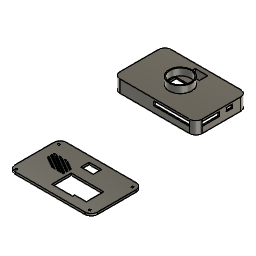
Camra_V1 v1 (Autodesk Fusion 360 design; units mm, degrees)
Autodesk Fusion 360 part; units mm, degrees
sketch "Boceto1" plane through (0, 0, 0) normal (0, 0, 1) x (1, 0, 0)
  line L0 (7, 0) -> (108, 0)
  line L1 (0, -7) -> (0, -63)
  line L2 (7, -70) -> (108, -70)
  line L3 (115, -63) -> (115, -7)
  arc A0 (7, 0) -> (0, -7) centre (7, -7) ccw
  arc A1 (0, -63) -> (7, -70) centre (7, -63) ccw
  arc A2 (108, -70) -> (115, -63) centre (108, -63) ccw
  arc A3 (115, -7) -> (108, 0) centre (108, -7) ccw
  line L4 (67.5, -3.5) -> (47.5, -3.5)
  line L5 (47.5, -3.5) -> (47.5, -17.5)
  line L6 (47.5, -17.5) -> (67.5, -17.5)
  line L7 (67.5, -17.5) -> (67.5, -3.5)
  circle A4 centre (4.1716, -4.1716) radius 2
  circle A5 centre (4.1716, -65.8284) radius 2
  circle A6 centre (108.8284, -63.8284) radius 2
  circle A7 centre (110.8284, -4.1716) radius 2
  line L8 (48.5, -4.5) -> (48.5, -16.5)
  line L9 (48.5, -16.5) -> (66.5, -16.5)
  line L10 (66.5, -16.5) -> (66.5, -4.5)
  line L11 (66.5, -4.5) -> (48.5, -4.5)
  arc A8 (117, -7) -> (108, 2) centre (108, -7) ccw
  line L12 (7, 2) -> (108, 2)
  arc A9 (7, 2) -> (-2, -7) centre (7, -7) ccw
  line L13 (-2, -7) -> (-2, -63)
  arc A10 (-2, -63) -> (7, -72) centre (7, -63) ccw
  line L14 (7, -72) -> (108, -72)
  arc A11 (108, -72) -> (117, -63) centre (108, -63) ccw
  line L15 (117, -63) -> (117, -7)
  arc A12 (0, -164.4825) -> (7, -171.4825) centre (7, -164.4825) ccw
  line L16 (66.5, -107.9825) -> (48.5, -107.9825)
  arc A13 (117, -108.4825) -> (108, -99.4825) centre (108, -108.4825) ccw
  circle A14 centre (108.8284, -167.311) radius 1.5
  circle A15 centre (110.8284, -107.6541) radius 1.5
  arc A16 (-2, -164.4825) -> (7, -173.4825) centre (7, -164.4825) ccw
  line L17 (48.5, -119.9825) -> (66.5, -119.9825)
  line L18 (67.5, -120.9825) -> (67.5, -106.9825)
  line L19 (67.5, -106.9825) -> (47.5, -106.9825)
  line L20 (47.5, -120.9825) -> (67.5, -120.9825)
  line L21 (47.5, -106.9825) -> (47.5, -120.9825)
  line L22 (7, -173.4825) -> (108, -173.4825)
  line L23 (7, -101.4825) -> (108, -101.4825)
  line L24 (7, -171.4825) -> (108, -171.4825)
  line L25 (-2, -108.4825) -> (-2, -164.4825)
  line L26 (0, -108.4825) -> (0, -164.4825)
  arc A17 (115, -108.4825) -> (108, -101.4825) centre (108, -108.4825) ccw
  circle A18 centre (4.1716, -169.311) radius 1.5
  arc A19 (108, -171.4825) -> (115, -164.4825) centre (108, -164.4825) ccw
  line L27 (115, -164.4825) -> (115, -108.4825)
  arc A20 (7, -99.4825) -> (-2, -108.4825) centre (7, -108.4825) ccw
  line L28 (48.5, -107.9825) -> (48.5, -119.9825)
  arc A21 (7, -101.4825) -> (0, -108.4825) centre (7, -108.4825) ccw
  arc A22 (108, -173.4825) -> (117, -164.4825) centre (108, -164.4825) ccw
  circle A23 centre (4.1716, -107.6541) radius 1.5
  line L29 (66.5, -119.9825) -> (66.5, -107.9825)
  line L30 (117, -164.4825) -> (117, -108.4825)
  line L31 (7, -99.4825) -> (108, -99.4825)
  circle A24 centre (57.5, -35) radius 16.5
  circle A25 centre (57.5, -35) radius 15
  line L32 (57.5, -29) -> (57.0394, -29)
  line L33 (57.5, -29) -> (58, -29)
  line L34 (58, -29) -> (68.4659, -29)
  line L35 (57.5, -29) -> (46.5341, -29)
  line L36 (57.5, -41) -> (68.4659, -41)
  line L37 (57.5, -41) -> (46.5341, -41)
  arc A26 (46.5341, -41) -> (68.4659, -41) centre (57.5, -35) ccw
  arc A27 (68.4659, -29) -> (46.5341, -29) centre (57.5, -35) ccw
  line L38 (68.4659, -29) -> (68.4659, -41)
  line L39 (46.5341, -29) -> (46.5341, -41)
  circle A28 centre (57.5, -35) radius 12.5081
  line L40 (12, -125) -> (40, -141)
  line L41 (12, -123) -> (43, -141)
  line L42 (15, -122) -> (44, -138.8387)
  line L43 (18.983, -122) -> (44, -136.526)
  line L44 (22.966, -122) -> (44, -134.2133)
  line L45 (12, -127.3035) -> (35.9689, -141)
  line L46 (12, -129.607) -> (31.9377, -141)
  line L47 (12, -131.9105) -> (27.9066, -141)
  line L48 (26.949, -122) -> (44, -131.9006)
  line L49 (12, -131.9105) -> (12, -129.607)
  line L50 (31.9377, -141) -> (27.9066, -141)
  line L51 (12, -127.3035) -> (12, -125)
  line L52 (12, -123) -> (12, -122)
  line L53 (44, -141) -> (43, -141)
  line L54 (40, -141) -> (35.9689, -141)
  line L55 (12, -122) -> (15, -122)
  line L56 (44, -138.8387) -> (44, -141)
  line L57 (44, -134.2133) -> (44, -136.526)
  line L58 (18.983, -122) -> (22.966, -122)
  line L59 (34.3764, -124) -> (42, -128.4266)
  line L60 (34.3764, -124) -> (30.932, -122)
  line L61 (42, -128.4266) -> (44, -129.5879)
  line L62 (30.932, -122) -> (26.949, -122)
  line L63 (44, -129.5879) -> (44, -131.9006)
  point P0 (115, 0)
  point P1 (0, -70)
  point P2 (0, -101.4825)
  point P3 (0, -101.4825)
  point P4 (0, -101.4825)
  point P5 (115, -101.4825)
  point P6 (0, -171.4825)
  dimension "d1" = 115
  dimension "d2" = 70
  dimension "d8" = 7
  dimension "d9" = 7
  dimension "d10" = 7
  dimension "d11" = 7
  dimension "d20" = 14
  dimension "d25" = 4
  dimension "d27" = 4
  dimension "d29" = 4
  dimension "d31" = 4
  dimension "d32" = -1
  dimension "d33" = -2
  dimension "d34" = -1
  dimension "d35" = -2
  dimension "d36" = 115
  dimension "d37" = 70
  dimension "d38" = 7
  dimension "d39" = 7
  dimension "d40" = 7
  dimension "d41" = 7
  dimension "d46" = 14
  dimension "d47" = 3
  dimension "d48" = 3
  dimension "d49" = 3
  dimension "d50" = 3
  dimension "d63" = 33
  dimension "d65" = 25
  constraint horizontal L0
  constraint perpendicular L0 L1
  constraint perpendicular L1 L2
  constraint perpendicular L0 L3
  constraint coincident origin L1
  constraint coincident origin L0
  constraint tangent L1 A0
  constraint tangent L0 A0
  constraint coincident P1 L2
  constraint coincident P1 L1
  constraint tangent L2 A1
  constraint tangent L1 A1
  constraint tangent L3 A2
  constraint tangent L2 A2
  constraint coincident P0 L3
  constraint coincident P0 L0
  constraint tangent L3 A3
  constraint tangent L0 A3
  constraint horizontal L4
  constraint vertical L5
  constraint horizontal L6
  constraint vertical L7
  constraint coincident P4 P3
  constraint horizontal L23
  constraint perpendicular L23 L26
  constraint perpendicular L24 L26
  constraint perpendicular L23 L27
  constraint coincident P4 L26
  constraint coincident P4 L23
  constraint tangent L26 A21
  constraint tangent L23 A21
  constraint coincident P6 L24
  constraint coincident P6 L26
  constraint tangent A12 L24
  constraint tangent A12 L26
  constraint tangent A19 L27
  constraint tangent L24 A19
  constraint coincident P5 L27
  constraint coincident P5 L23
  constraint tangent A17 L27
  constraint tangent L23 A17
  constraint horizontal L19
  constraint vertical L21
  constraint horizontal L20
  constraint vertical L18
  constraint concentric A24 A25
  constraint concentric A25 A26
  constraint coincident L34.end A26
  constraint concentric A26 A27
  constraint perpendicular L36 L38
  constraint perpendicular L37 L39
  constraint concentric A26 A28
  constraint coincident L40.end L53
  constraint parallel L41 L42
  constraint coincident L43.start L55
  constraint coincident L44.start L55
  constraint coincident L46.end L53
  constraint coincident L48.start L55
  constraint collinear L49 L51
  constraint collinear L50 L53
  constraint collinear L51 L52
  constraint collinear L53 L54
  constraint collinear L55 L58
  constraint parallel L59 L60
  constraint parallel L59 L61
  constraint horizontal L62
  constraint vertical L63
  measures "d1" distance of origin P0
  measures "d2" distance of origin P1
  measures "d8" radius of A0
  measures "d9" radius of A1
  measures "d10" radius of A2
  measures "d11" radius of A3
  measures "d20" distance of L4.start L6.end
  measures "d25" diameter of A4
  measures "d27" diameter of A5
  measures "d29" diameter of A6
  measures "d31" diameter of A7
  measures "d36" distance of P4 P5
  measures "d37" distance of P4 P6
  measures "d38" radius of A21
  measures "d39" radius of A12
  measures "d40" radius of A19
  measures "d41" radius of A17
  measures "d46" distance of L18.start L18.end
  measures "d47" diameter of A23
  measures "d48" diameter of A18
  measures "d49" diameter of A14
  measures "d50" diameter of A15
  measures "d63" diameter of A24
  measures "d65" diameter of A26
extrude "Extruir1" add sketch "Boceto1" along normal blind 3 contours L0 L1 L2 L3 A0 A1 A2 A3 | L4 L5 L6 L7 | A4 | A5 | A6 | A7 | A8 L12 A9 L13 A10 L14 A11 L15 | A24 | A25 | L32 L33 L34 L35 L36 L37 L38 L39 | L32 L33 L34 L35 A27 | L36 L37 A26 | A28 makes body 1
extrude "Extruir2" add sketch "Boceto1" along normal blind 18 separate body contours A8 L12 A9 L13 A10 L14 A11 L15 makes body 2
sketch "Boceto2" plane through (0, 0, 3) normal (0, 0, 1) x (-1, 0, 0)
  line L0 (-48.5, 4.5) -> (-66.5, 4.5)
  line L1 (-66.5, 4.5) -> (-66.5, 16.5)
  line L2 (-66.5, 16.5) -> (-48.5, 16.5)
  line L3 (-48.5, 16.5) -> (-48.5, 4.5)
  arc A0 (-7, -2) -> (2, 7) centre (-7, 7) ccw
  line L4 (2, 7) -> (2, 63)
  arc A1 (2, 63) -> (-7, 72) centre (-7, 63) ccw
  line L5 (-7, 72) -> (-108, 72)
  arc A2 (-108, 72) -> (-117, 63) centre (-108, 63) ccw
  line L6 (-117, 63) -> (-117, 7)
  arc A3 (-117, 7) -> (-108, -2) centre (-108, 7) ccw
  line L7 (-108, -2) -> (-7, -2)
  line L8 (-46.5405, 21.9969) -> (-68.4761, 21.9969)
  line L9 (-70.4761, 23.9969) -> (-70.4761, 46)
  line L10 (-68.4761, 48) -> (-46.5405, 48)
  line L11 (-44.5405, 46) -> (-44.5405, 23.9969)
  arc A4 (-46.5405, 21.9969) -> (-44.5405, 23.9969) centre (-46.5405, 23.9969) ccw
  arc A5 (-70.4761, 23.9969) -> (-68.4761, 21.9969) centre (-68.4761, 23.9969) ccw
  arc A6 (-68.4761, 48) -> (-70.4761, 46) centre (-68.4761, 46) ccw
  arc A7 (-44.5405, 46) -> (-46.5405, 48) centre (-46.5405, 46) ccw
  circle A8 centre (-46.5405, 23.9969) radius 1.75
  circle A9 centre (-46.5405, 46) radius 1.75
  line L12 (-57, 29) -> (-57.2613, 29)
  line L13 (-57.2613, 29) -> (-70.4761, 29)
  line L14 (-57, 29) -> (-44.5405, 29)
  line L15 (-57.0405, 41) -> (-70.4761, 41)
  line L16 (-57.0405, 41) -> (-44.5405, 41)
  dimension "d55" = 2
  dimension "d56" = 2
  dimension "d57" = 2
  dimension "d58" = 2
  dimension "d70" = 3.5
  dimension "d71" = 3.5
  constraint horizontal L8
  constraint perpendicular L8 L9
  constraint perpendicular L9 L10
  constraint perpendicular L10 L11
  constraint tangent L11 A4
  constraint tangent L8 A4
  constraint tangent L8 A5
  constraint tangent L9 A5
  constraint tangent L9 A6
  constraint tangent L10 A6
  constraint tangent L11 A7
  constraint tangent L10 A7
  constraint concentric A4 A8
  constraint concentric A7 A9
  constraint perpendicular L11 L12
  constraint coincident L9 L13.end
  constraint perpendicular L9 L13
  constraint coincident L11 L14.end
  constraint perpendicular L11 L14
  constraint coincident L9 L15.end
  constraint perpendicular L9 L15
  constraint coincident L11 L16.end
  constraint perpendicular L11 L16
  measures "d55" radius of A4
  measures "d56" radius of A5
  measures "d57" radius of A6
  measures "d58" radius of A7
  measures "d70" diameter of A8
  measures "d71" diameter of A9
extrude "Extruir3" cut sketch "Boceto2" against normal blind 1 contours L8 L9 L11 A4 A5 L12 L13 L14 | L9 L11 L12 L13 L14 L15 L16 | L9 L10 L11 A6 A7 L15 L16 | A8 | A9 bodies 1
extrude "Extruir5" add sketch "Boceto1" along normal blind 1 separate body contours A25 | L32 L33 L34 L35 L36 L37 L38 L39 | A28 makes body 3
extrude "Extruir6" add sketch "Boceto1" along normal blind 1 contours A24 bodies 1 3
extrude "Extruir7" cut sketch "Boceto2" against normal blind 2 contours A8 bodies 1
extrude "Extruir8" cut sketch "Boceto2" against normal blind 2 contours A9 bodies 1
extrude "Extruir9" cut sketch "Boceto2" against normal blind 4 contours L9 L11 L12 L13 L14 L15 L16 bodies 1
extrude "Extruir10" add sketch "Boceto1" against normal blind 10 contours A24 bodies 1
extrude "Extruir11" add sketch "Boceto1" along normal blind 18 separate body contours L4 L5 L6 L7 makes body 4
sketch "Boceto3" plane through (0, 2, 0) normal (0, 1, 0) x (-1, 0, 0)
  line L0 (-108, 0) -> (-7, 0)
  line L1 (-7, 0) -> (-7, 18)
  line L2 (-7, 18) -> (-108, 18)
  line L3 (-108, 18) -> (-108, 0)
  circle A0 centre (-95, 9) radius 4.75
  dimension "d87" = 9.5
  measures "d87" diameter of A0
extrude "Extruir12" cut sketch "Boceto3" against normal blind 3 contours A0 bodies 2
sketch "Boceto4" plane through (0, 0, 3) normal (0, 0, 1) x (-1, 0, 0)
  line L0 (-44.5405, 46) -> (-44.5405, 23.9969)
  arc A0 (-46.5405, 21.9969) -> (-44.5405, 23.9969) centre (-46.5405, 23.9969) ccw
  line L1 (-46.5405, 21.9969) -> (-68.4761, 21.9969)
  arc A1 (-70.4761, 23.9969) -> (-68.4761, 21.9969) centre (-68.4761, 23.9969) ccw
  line L2 (-70.4761, 23.9969) -> (-70.4761, 46)
  arc A2 (-68.4761, 48) -> (-70.4761, 46) centre (-68.4761, 46) ccw
  line L3 (-68.4761, 48) -> (-46.5405, 48)
  arc A3 (-44.5405, 46) -> (-46.5405, 48) centre (-46.5405, 46) ccw
  line L4 (-48.5, 4.5) -> (-66.5, 4.5)
  line L5 (-66.5, 4.5) -> (-66.5, 16.5)
  line L6 (-66.5, 16.5) -> (-48.5, 16.5)
  line L7 (-48.5, 16.5) -> (-48.5, 4.5)
  arc A4 (-7, -2) -> (2, 7) centre (-7, 7) ccw
  line L8 (2, 7) -> (2, 63)
  arc A5 (2, 63) -> (-7, 72) centre (-7, 63) ccw
  line L9 (-7, 72) -> (-108, 72)
  arc A6 (-108, 72) -> (-117, 63) centre (-108, 63) ccw
  line L10 (-117, 63) -> (-117, 7)
  arc A7 (-117, 7) -> (-108, -2) centre (-108, 7) ccw
  line L11 (-108, -2) -> (-7, -2)
  line L12 (-42, 68.1443) -> (-39, 68.1443)
  line L13 (-39, 68.1443) -> (-68.2633, 68.1443)
  line L14 (-68.2633, 68.1443) -> (-3.2633, 68.1443)
  line L15 (-3.2633, 68.1443) -> (-3.2633, 38.1443)
  line L16 (-3.2633, 38.1443) -> (-68.2633, 38.1443)
  line L17 (-68.2633, 38.1443) -> (-68.2633, 68.1443)
  circle A8 centre (-4, 4) radius 2.2361
  circle A9 centre (-111, 4) radius 2.2361
  circle A10 centre (-108.8284, 63.8284) radius 2
  circle A11 centre (-108.8284, 63.8284) radius 2
  circle A12 centre (-4, 4) radius 3
  circle A13 centre (-111, 4) radius 3
  line L18 (-71.6644, 9.3288) -> (-71.6644, 59.3288)
  line L19 (-71.6644, 9.3288) -> (-111.6644, 9.3288)
  line L20 (-71.6644, 59.3288) -> (-111.6644, 59.3288)
  line L21 (-111.6644, 59.3288) -> (-111.6644, 9.3288)
  dimension "d99" = 65
  dimension "d100" = 30
  dimension "d121" = 6
  dimension "d129" = 6
  dimension "d142" = 50
  dimension "d143" = 40
  constraint horizontal L12
  constraint parallel L12 L13
  constraint parallel L13 L14
  constraint perpendicular L14 L15
  constraint perpendicular L2 L16
  constraint perpendicular L14 L17
  constraint concentric A10 A11
  constraint concentric A8 A12
  constraint concentric A9 A13
  constraint parallel L7 L18
  constraint perpendicular L18 L19
  constraint perpendicular L18 L20
  constraint perpendicular L19 L21
  measures "d99" distance of L13.end L14.end
  measures "d100" distance of L14.end L15.end
  measures "d121" diameter of A12
  measures "d129" diameter of A13
  measures "d142" distance of L18.start L18.end
  measures "d143" distance of L18.start L19.end
sketch "Boceto5" plane through (0, 0, 0) normal (1, 0, 0) x (0, 1, 0)
  line L0 (-63, 0) -> (-7, 0)
  line L1 (-7, 0) -> (-7, 18)
  line L2 (-7, 18) -> (-63, 18)
  line L3 (-63, 18) -> (-63, 0)
  line L4 (-63, 3) -> (-63, 9)
  line L5 (-63, 9) -> (-38, 9)
  line L6 (-38, 9) -> (-38, 3)
  line L7 (-38, 3) -> (-63, 3)
  dimension "d90" = 6
  dimension "d91" = 25
  constraint coincident L3 L4.start
  constraint perpendicular L4 L5
  constraint perpendicular L5 L6
  constraint perpendicular L3 L7
  measures "d90" distance of L4.start L4.end
  measures "d91" distance of L4.end L5.end
extrude "Extruir13" cut sketch "Boceto5" against normal blind 2 contours L3 L4 L5 L6 L7 bodies 2
sketch "Boceto6" plane through (0, -70, 0) normal (0, 1, 0) x (-1, 0, 0)
  line L0 (-108, 0) -> (-7, 0)
  line L1 (-7, 0) -> (-7, 18)
  line L2 (-7, 18) -> (-108, 18)
  line L3 (-108, 18) -> (-108, 0)
  line L4 (-7, 3) -> (-7, 9)
  line L5 (-7, 9) -> (-59, 9)
  line L6 (-59, 9) -> (-59, 3)
  line L7 (-59, 3) -> (-7, 3)
  dimension "d94" = 6
  dimension "d96" = 52
  constraint coincident L1 L4.start
  constraint perpendicular L2 L4
  constraint perpendicular L1 L5
  constraint perpendicular L5 L6
  constraint perpendicular L4 L7
  measures "d94" distance of L4.start L4.end
  measures "d96" distance of L4.end L5.end
extrude "Extruir14" cut sketch "Boceto6" against normal blind 12 contours L1 L4 L5 L6 L7 bodies 2
sketch "Boceto7" plane through (0, 0, 0) normal (1, 0, 0) x (0, 1, 0)
  line L0 (-38, 3) -> (-63, 3)
  line L1 (-63, 3) -> (-63, 0)
  line L2 (-63, 0) -> (-7, 0)
  line L3 (-7, 0) -> (-7, 18)
  line L4 (-7, 18) -> (-63, 18)
  line L5 (-63, 18) -> (-63, 9)
  line L6 (-63, 9) -> (-38, 9)
  line L7 (-38, 9) -> (-38, 3)
  line L8 (-38, 9) -> (-28, 9)
  line L9 (-28, 9) -> (-28, 3)
  line L10 (-28, 3) -> (-28, 8)
  line L11 (-28, 8) -> (-19, 8)
  line L12 (-19, 8) -> (-19, 3)
  line L13 (-19, 3) -> (-28, 3)
  dimension "d103" = 10
  dimension "d104" = 5
  dimension "d105" = 9
  constraint coincident L6.end L7.start
  constraint perpendicular L7 L8
  constraint perpendicular L8 L9
  constraint parallel L9 L10
  constraint perpendicular L9 L11
  constraint perpendicular L11 L12
  constraint perpendicular L9 L13
  measures "d103" distance of L6.end L8.end
  measures "d104" distance of L9.end L10.end
  measures "d105" distance of L10.end L11.end
extrude "Extruir16" cut sketch "Boceto7" against normal blind 3 contours L9 L10 L11 L12 L13 bodies 2
sketch "Boceto8" plane through (0, 0, 3) normal (0, 0, 1) x (-1, 0, 0)
  line L0 (-44.5405, 46) -> (-44.5405, 23.9969)
  arc A0 (-46.5405, 21.9969) -> (-44.5405, 23.9969) centre (-46.5405, 23.9969) ccw
  line L1 (-46.5405, 21.9969) -> (-68.4761, 21.9969)
  arc A1 (-70.4761, 23.9969) -> (-68.4761, 21.9969) centre (-68.4761, 23.9969) ccw
  line L2 (-70.4761, 23.9969) -> (-70.4761, 46)
  arc A2 (-68.4761, 48) -> (-70.4761, 46) centre (-68.4761, 46) ccw
  line L3 (-68.4761, 48) -> (-46.5405, 48)
  arc A3 (-44.5405, 46) -> (-46.5405, 48) centre (-46.5405, 46) ccw
  line L4 (-48.5, 4.5) -> (-66.5, 4.5)
  line L5 (-66.5, 4.5) -> (-66.5, 16.5)
  line L6 (-66.5, 16.5) -> (-48.5, 16.5)
  line L7 (-48.5, 16.5) -> (-48.5, 4.5)
  arc A4 (-7, -2) -> (2, 7) centre (-7, 7) ccw
  line L8 (2, 7) -> (2, 63)
  arc A5 (2, 63) -> (-7, 72) centre (-7, 63) ccw
  line L9 (-7, 72) -> (-108, 72)
  arc A6 (-108, 72) -> (-117, 63) centre (-108, 63) ccw
  line L10 (-117, 63) -> (-117, 7)
  arc A7 (-117, 7) -> (-108, -2) centre (-108, 7) ccw
  line L11 (-108, -2) -> (-7, -2)
  line L12 (0, 20) -> (-45, 20)
  circle A8 centre (-108.7791, 63.7758) radius 3
  circle A9 centre (-111, 4) radius 3
  circle A10 centre (-4, 4) radius 3
  dimension "d108" = 45
  dimension "d110" = 6
  dimension "d111" = 6
  dimension "d112" = 6
  constraint horizontal L12
  measures "d108" distance of L12.start L12.end
  measures "d110" diameter of A8
  measures "d111" diameter of A9
  measures "d112" diameter of A10
extrude "Extruir17" add sketch "Boceto8" along normal blind 12 contours A8 bodies 1
sketch "Boceto9" plane through (0, 0, 15) normal (0, 0, 1) x (-1, 0, 0)
  circle A0 centre (-108.7791, 63.7758) radius 3
  circle A1 centre (-108.7791, 63.7758) radius 2
  dimension "d115" = 4
  constraint concentric A0 A1
  measures "d115" diameter of A1
extrude "Extruir18" cut sketch "Boceto9" against normal blind 3 contours A1 bodies 1
extrude "Extruir20" cut sketch "Boceto4" along normal blind 13 contours A8 | A12 bodies 2
extrude "Extruir21" add sketch "Boceto4" along normal blind 13 contours A8 | A12 bodies 1 2
sketch "Boceto11" plane through (0, 0, 16) normal (0, 0, 1) x (-1, 0, 0)
  arc A0 (-3.2339, 1.0995) -> (-1.0995, 3.2339) centre (-7, 7) ccw
  arc A1 (-1.0995, 3.2339) -> (-3.2339, 1.0995) centre (-4, 4) ccw
  circle A2 centre (-4, 4) radius 2
  dimension "d126" = 4
  constraint concentric A1 A2
  measures "d126" diameter of A2
extrude "Extruir22" cut sketch "Boceto11" against normal blind 3 contours A2 bodies 1
extrude "Extruir23" cut sketch "Boceto4" along normal blind 13 contours A9 | A13 bodies 1
extrude "Extruir24" add sketch "Boceto4" along normal blind 13 contours A9 | A13 bodies 1
sketch "Boceto12" plane through (0, 0, 16) normal (0, 0, 1) x (-1, 0, 0)
  arc A0 (-113.9005, 3.2339) -> (-111.7661, 1.0995) centre (-108, 7) ccw
  arc A1 (-111.7661, 1.0995) -> (-113.9005, 3.2339) centre (-111, 4) ccw
  circle A2 centre (-111, 4) radius 2
  dimension "d134" = 4
  constraint concentric A1 A2
  measures "d134" diameter of A2
extrude "Extruir25" cut sketch "Boceto12" against normal blind 3 contours A2 bodies 1
sketch "Boceto13" plane through (115, 0, 0) normal (-1, 0, 0) x (0, -1, 0)
  line L0 (7, 3) -> (63, 3)
  line L1 (63, 3) -> (63, 18)
  line L2 (63, 18) -> (7, 18)
  line L3 (7, 18) -> (7, 3)
  line L4 (7, 3) -> (7, 10.5)
  line L5 (9.6121, 10.5) -> (9.6121, 8.5)
  line L6 (18.6121, 10.5) -> (18.6121, 12.5)
  line L7 (9.6121, 8.5) -> (18.6121, 8.5)
  line L8 (18.6121, 8.5) -> (18.6121, 12.5)
  line L9 (18.6121, 12.5) -> (9.6121, 12.5)
  line L10 (9.6121, 12.5) -> (9.6121, 8.5)
  dimension "d137" = 9
  dimension "d138" = 2
  dimension "d139" = 2
  constraint coincident L0.start L3.end
  constraint midpoint L3 L4.end
  constraint horizontal L7
  constraint vertical L8
  constraint horizontal L9
  constraint vertical L10
  measures "d137" distance of L5.start L6.start
  measures "d138" distance of L5.start L5.end
  measures "d139" distance of L6.start L6.end
extrude "Extruir26" cut sketch "Boceto13" against normal blind 8 contours L5 L6 L7 L8 L9 L10 bodies 1
extrude "Extruir28" add sketch "Boceto1" along normal blind 3 separate body contours A12 L23 L24 L26 A17 A18 A19 L27 A21 | A12 A18 | A12 A18 | A13 A16 L22 L25 A20 A22 L30 L31 | A14 | A15 | L18 L19 L20 L21 | A23 | L40 L45 L51 L54 | L41 L42 L52 L53 L55 L56 | L43 L44 L57 L58 | L46 L47 L49 L50 | L48 L59 L60 L61 L62 L63 makes body 5
sketch "Boceto14" plane through (0, 0, 3) normal (0, 0, 1) x (-1, 0, 0)
  line L0 (-66.5, 107.9825) -> (-66.5, 119.9825)
  line L1 (-66.5, 119.9825) -> (-48.5, 119.9825)
  line L2 (-48.5, 119.9825) -> (-48.5, 107.9825)
  line L3 (-48.5, 107.9825) -> (-66.5, 107.9825)
  line L4 (2, 108.4825) -> (2, 164.4825)
  arc A0 (2, 164.4825) -> (-7, 173.4825) centre (-7, 164.4825) ccw
  line L5 (-7, 173.4825) -> (-108, 173.4825)
  arc A1 (-108, 173.4825) -> (-117, 164.4825) centre (-108, 164.4825) ccw
  line L6 (-117, 164.4825) -> (-117, 108.4825)
  arc A2 (-117, 108.4825) -> (-108, 99.4825) centre (-108, 108.4825) ccw
  line L7 (-108, 99.4825) -> (-7, 99.4825)
  arc A3 (-7, 99.4825) -> (2, 108.4825) centre (-7, 108.4825) ccw
  line L8 (-96, 154.4825) -> (-96, 134.4825)
  line L9 (-96, 134.4825) -> (-49, 134.4825)
  line L10 (-49, 134.4825) -> (-49, 162.4825)
  line L11 (-96, 134.4825) -> (-96, 159.4825)
  line L12 (-96, 159.4825) -> (-79, 159.4825)
  line L13 (-49, 162.4825) -> (-79, 162.4825)
  line L14 (-79, 162.4825) -> (-79, 159.4825)
  dimension "d151" = 47
  dimension "d152" = 28
  dimension "d154" = 25
  constraint perpendicular L8 L9
  constraint perpendicular L9 L10
  constraint perpendicular L9 L11
  constraint perpendicular L11 L12
  constraint perpendicular L10 L13
  measures "d151" distance of L8.end L9.end
  measures "d152" distance of L9.end L10.end
  measures "d154" distance of L8.end L11.end
extrude "Extruir29" cut sketch "Boceto14" against normal blind 6 contours L8 L9 L10 L11 L12 L13 L14 bodies 5
extrude "Extruir30" cut sketch "Boceto1" along normal blind 3 contours A23 bodies 5
extrude "Extruir31" cut sketch "Boceto1" along normal blind 5 contours A12 A18 picked at (3.9622, -169.6917) bodies 5
extrude "Extruir32" cut sketch "Boceto1" along normal blind 9 contours A14 bodies 5
extrude "Extruir33" cut sketch "Boceto1" along normal blind 13 contours A15 bodies 5
extrude "Extruir34" cut sketch "Boceto1" along normal blind 4 contours L40 L45 L51 L54 | L41 L42 L52 L53 L55 L56 | L43 L44 L57 L58 | L46 L47 L49 L50 | L48 L59 L60 L61 L62 L63 bodies 5
combine "Combinar1" operation add target body 1 tool bodies 4
move_body "Desplazar1" bodies 1 to x (-1, 0, 0) y (0, 1, 0) z (0, 0, -1) at (-4, 0, -20)
move_body "Desplazar2" bodies 1 to x (1, 0, 0) y (0, 1, 0) z (0, 0, 1) at (119.1989, 49.9549, 63.9258)
